Autodesk Fusion 360 part; units mm, degrees
(part 5 of 11)
  arc A140 (-29.854, -24.6972) -> (-30.0927, -24.4471) centre (-30.104, -24.6968) ccw construction
  arc A141 (-29.854, -24.6972) -> (-29.853, -24.8125) centre (-23.9648, -24.7074) ccw construction
  arc A142 (-30.0877, -25.0665) -> (-29.853, -24.8125) centre (-30.103, -24.8169) ccw construction
  line L76 (-30.0877, -25.0665) -> (-30.1561, -25.0707) construction
  spline S70 degree 5 poles (-30.1561, -25.0707) (-30.1588, -25.0708) (-30.1643, -25.0712) (-30.1725, -25.072) (-30.1834, -25.0735) (-30.197, -25.0758) (-30.2105, -25.0785) (-30.224, -25.0814) (-30.2375, -25.0845) (-30.251, -25.0877) (-30.2645, -25.091) (-30.278, -25.0944) (-30.2915, -25.098) (-30.3049, -25.1017) (-30.3183, -25.1056) (-30.3317, -25.1097) (-30.3451, -25.114) (-30.3585, -25.1183) (-30.3719, -25.1228) (-30.3852, -25.1274) (-30.3986, -25.1321) (-30.4119, -25.1369) (-30.4252, -25.1418) (-30.4385, -25.1469) (-30.4518, -25.152) (-30.4651, -25.1573) (-30.4783, -25.1626) (-30.4915, -25.1681) (-30.5048, -25.1737) (-30.518, -25.1793) (-30.5312, -25.1851) (-30.5443, -25.1909) (-30.5575, -25.1969) (-30.5707, -25.2029) (-30.5838, -25.2091) (-30.5969, -25.2153) (-30.61, -25.2216) (-30.6231, -25.228) (-30.6362, -25.2345) (-30.6492, -25.2411) (-30.6623, -25.2478) (-30.6753, -25.2545) (-30.6883, -25.2613) (-30.7013, -25.2683) (-30.7143, -25.2753) (-30.7272, -25.2824) (-30.7402, -25.2895) (-30.7531, -25.2968) (-30.766, -25.3041) (-30.7789, -25.3115) (-30.7918, -25.319) (-30.8046, -25.3266) (-30.8175, -25.3342) (-30.8303, -25.3419) (-30.8431, -25.3497) (-30.8559, -25.3576) (-30.8686, -25.3655) (-30.8814, -25.3735) (-30.8941, -25.3816) (-30.9068, -25.3898) (-30.9195, -25.398) (-30.9322, -25.4064) (-30.9449, -25.4147) (-30.9575, -25.4232) (-30.9701, -25.4317) (-30.9827, -25.4403) (-30.9953, -25.449) (-31.0079, -25.4578) (-31.0204, -25.4666) (-31.033, -25.4755) (-31.0455, -25.4844) (-31.0555, -25.4916) (-31.0629, -25.4971) (-31.0679, -25.5007) (-31.0704, -25.5025) knots 0 0 0 0 0 0 0.01428571 0.02857143 0.04285714 0.05714286 0.07142857 0.08571429 0.1 0.11428571 0.12857143 0.14285714 0.15714286 0.17142857 0.18571429 0.2 0.21428571 0.22857143 0.24285714 0.25714286 0.27142857 0.28571429 0.3 0.31428571 0.32857143 0.34285714 0.35714286 0.37142857 0.38571429 0.4 0.41428571 0.42857143 0.44285714 0.45714286 0.47142857 0.48571429 0.5 0.51428571 0.52857143 0.54285714 0.55714286 0.57142857 0.58571429 0.6 0.61428571 0.62857143 0.64285714 0.65714286 0.67142857 0.68571429 0.7 0.71428571 0.72857143 0.74285714 0.75714286 0.77142857 0.78571429 0.8 0.81428571 0.82857143 0.84285714 0.85714286 0.87142857 0.88571429 0.9 0.91428571 0.92857143 0.94285714 0.95714286 0.97142857 0.98571429 1 1 1 1 1 1 construction
  arc A143 (-31.0704, -25.5025) -> (-31.0159, -25.8922) centre (-23.9648, -24.7074) ccw construction
  spline S71 degree 5 poles (-31.0159, -25.8922) (-31.013, -25.8933) (-31.0072, -25.8955) (-30.9985, -25.8986) (-30.9869, -25.9028) (-30.9725, -25.908) (-30.958, -25.9131) (-30.9435, -25.9182) (-30.929, -25.9231) (-30.9145, -25.928) (-30.9001, -25.9328) (-30.8856, -25.9376) (-30.8711, -25.9422) (-30.8566, -25.9468) (-30.8422, -25.9513) (-30.8277, -25.9558) (-30.8132, -25.9601) (-30.7988, -25.9644) (-30.7843, -25.9687) (-30.7698, -25.9728) (-30.7554, -25.9768) (-30.7409, -25.9808) (-30.7265, -25.9847) (-30.712, -25.9886) (-30.6976, -25.9923) (-30.6832, -25.996) (-30.6687, -25.9996) (-30.6543, -26.0031) (-30.6399, -26.0065) (-30.6255, -26.0098) (-30.6111, -26.0131) (-30.5967, -26.0163) (-30.5823, -26.0193) (-30.5679, -26.0223) (-30.5535, -26.0253) (-30.5392, -26.0281) (-30.5248, -26.0308) (-30.5104, -26.0335) (-30.4961, -26.0361) (-30.4818, -26.0386) (-30.4674, -26.0409) (-30.4531, -26.0432) (-30.4388, -26.0454) (-30.4245, -26.0476) (-30.4103, -26.0496) (-30.396, -26.0515) (-30.3817, -26.0533) (-30.3675, -26.055) (-30.3533, -26.0567) (-30.3391, -26.0582) (-30.3249, -26.0596) (-30.3107, -26.0609) (-30.2965, -26.0621) (-30.2824, -26.0632) (-30.2682, -26.0641) (-30.2541, -26.065) (-30.24, -26.0657) (-30.2259, -26.0664) (-30.2119, -26.0669) (-30.1978, -26.0673) (-30.1838, -26.0676) (-30.1698, -26.0677) (-30.1558, -26.0676) (-30.1419, -26.0673) (-30.128, -26.0669) (-30.1141, -26.0663) (-30.1003, -26.0657) (-30.0865, -26.065) (-30.0727, -26.0641) (-30.0589, -26.063) (-30.0452, -26.0615) (-30.0343, -26.0599) (-30.0262, -26.0584) (-30.0209, -26.0573) (-30.0182, -26.0567) knots -1 -1 -1 -1 -1 -1 -0.98571429 -0.97142857 -0.95714286 -0.94285714 -0.92857143 -0.91428571 -0.9 -0.88571429 -0.87142857 -0.85714286 -0.84285714 -0.82857143 -0.81428571 -0.8 -0.78571429 -0.77142857 -0.75714286 -0.74285714 -0.72857143 -0.71428571 -0.7 -0.68571429 -0.67142857 -0.65714286 -0.64285714 -0.62857143 -0.61428571 -0.6 -0.58571429 -0.57142857 -0.55714286 -0.54285714 -0.52857143 -0.51428571 -0.5 -0.48571429 -0.47142857 -0.45714286 -0.44285714 -0.42857143 -0.41428571 -0.4 -0.38571429 -0.37142857 -0.35714286 -0.34285714 -0.32857143 -0.31428571 -0.3 -0.28571429 -0.27142857 -0.25714286 -0.24285714 -0.22857143 -0.21428571 -0.2 -0.18571429 -0.17142857 -0.15714286 -0.14285714 -0.12857143 -0.11428571 -0.1 -0.08571429 -0.07142857 -0.05714286 -0.04285714 -0.02857143 -0.01428571 0 0 0 0 0 0 construction
  line L77 (-30.0182, -26.0567) -> (-29.9513, -26.042) construction
  arc A144 (-29.6559, -26.2218) -> (-29.9513, -26.042) centre (-29.8975, -26.2861) ccw construction
  arc A145 (-29.6559, -26.2218) -> (-29.6252, -26.3329) centre (-23.9648, -24.7074) ccw construction
  arc A146 (-29.7862, -26.639) -> (-29.6252, -26.3329) centre (-29.8655, -26.4019) ccw construction
  line L78 (-29.7862, -26.639) -> (-29.8511, -26.6607) construction
  spline S72 degree 5 poles (-29.8511, -26.6607) (-29.8537, -26.6616) (-29.8589, -26.6634) (-29.8666, -26.6663) (-29.8768, -26.6705) (-29.8893, -26.6763) (-29.9016, -26.6824) (-29.9139, -26.6887) (-29.9262, -26.6952) (-29.9384, -26.7018) (-29.9506, -26.7084) (-29.9627, -26.7152) (-29.9748, -26.7221) (-29.9868, -26.7292) (-29.9988, -26.7365) (-30.0107, -26.7439) (-30.0225, -26.7515) (-30.0343, -26.7592) (-30.046, -26.767) (-30.0578, -26.7748) (-30.0694, -26.7828) (-30.0811, -26.7909) (-30.0926, -26.7991) (-30.1042, -26.8074) (-30.1157, -26.8158) (-30.1271, -26.8243) (-30.1385, -26.8329) (-30.1499, -26.8417) (-30.1612, -26.8505) (-30.1725, -26.8593) (-30.1838, -26.8683) (-30.195, -26.8774) (-30.2062, -26.8865) (-30.2173, -26.8958) (-30.2284, -26.9051) (-30.2395, -26.9145) (-30.2505, -26.924) (-30.2615, -26.9336) (-30.2724, -26.9432) (-30.2833, -26.953) (-30.2942, -26.9628) (-30.305, -26.9727) (-30.3158, -26.9826) (-30.3266, -26.9927) (-30.3373, -27.0028) (-30.348, -27.013) (-30.3586, -27.0233) (-30.3692, -27.0336) (-30.3798, -27.0441) (-30.3904, -27.0545) (-30.4009, -27.0651) (-30.4113, -27.0757) (-30.4217, -27.0864) (-30.4321, -27.0972) (-30.4425, -27.1081) (-30.4528, -27.119) (-30.4631, -27.1299) (-30.4733, -27.141) (-30.4835, -27.1521) (-30.4937, -27.1633) (-30.5038, -27.1745) (-30.5139, -27.1859) (-30.524, -27.1972) (-30.534, -27.2087) (-30.544, -27.2202) (-30.5539, -27.2318) (-30.5638, -27.2434) (-30.5737, -27.2551) (-30.5835, -27.2668) (-30.5933, -27.2787) (-30.6031, -27.2906) (-30.6109, -27.3001) (-30.6167, -27.3073) (-30.6206, -27.3121) (-30.6225, -27.3145) knots 0 0 0 0 0 0 0.01428571 0.02857143 0.04285714 0.05714286 0.07142857 0.08571429 0.1 0.11428571 0.12857143 0.14285714 0.15714286 0.17142857 0.18571429 0.2 0.21428571 0.22857143 0.24285714 0.25714286 0.27142857 0.28571429 0.3 0.31428571 0.32857143 0.34285714 0.35714286 0.37142857 0.38571429 0.4 0.41428571 0.42857143 0.44285714 0.45714286 0.47142857 0.48571429 0.5 0.51428571 0.52857143 0.54285714 0.55714286 0.57142857 0.58571429 0.6 0.61428571 0.62857143 0.64285714 0.65714286 0.67142857 0.68571429 0.7 0.71428571 0.72857143 0.74285714 0.75714286 0.77142857 0.78571429 0.8 0.81428571 0.82857143 0.84285714 0.85714286 0.87142857 0.88571429 0.9 0.91428571 0.92857143 0.94285714 0.95714286 0.97142857 0.98571429 1 1 1 1 1 1 construction
  arc A147 (-30.6225, -27.3145) -> (-30.469, -27.6768) centre (-23.9648, -24.7074) ccw construction
  spline S73 degree 5 poles (-30.469, -27.6768) (-30.4659, -27.6771) (-30.4598, -27.6777) (-30.4505, -27.6785) (-30.4383, -27.6796) (-30.4229, -27.6808) (-30.4076, -27.682) (-30.3923, -27.6831) (-30.3771, -27.6842) (-30.3618, -27.6851) (-30.3466, -27.6861) (-30.3314, -27.6869) (-30.3162, -27.6876) (-30.301, -27.6883) (-30.2859, -27.689) (-30.2707, -27.6895) (-30.2556, -27.69) (-30.2405, -27.6904) (-30.2255, -27.6907) (-30.2104, -27.691) (-30.1954, -27.6911) (-30.1804, -27.6912) (-30.1655, -27.6913) (-30.1505, -27.6912) (-30.1356, -27.6911) (-30.1207, -27.6909) (-30.1059, -27.6906) (-30.091, -27.6903) (-30.0762, -27.6899) (-30.0614, -27.6894) (-30.0467, -27.6888) (-30.0319, -27.6881) (-30.0172, -27.6874) (-30.0026, -27.6866) (-29.9879, -27.6857) (-29.9733, -27.6847) (-29.9587, -27.6836) (-29.9442, -27.6825) (-29.9297, -27.6812) (-29.9152, -27.6799) (-29.9007, -27.6785) (-29.8863, -27.677) (-29.8719, -27.6755) (-29.8576, -27.6738) (-29.8433, -27.6721) (-29.829, -27.6702) (-29.8147, -27.6683) (-29.8005, -27.6663) (-29.7864, -27.6642) (-29.7722, -27.6619) (-29.7582, -27.6596) (-29.7441, -27.6572) (-29.7301, -27.6547) (-29.7162, -27.6521) (-29.7023, -27.6494) (-29.6884, -27.6465) (-29.6746, -27.6436) (-29.6608, -27.6406) (-29.6471, -27.6375) (-29.6334, -27.6342) (-29.6198, -27.6308) (-29.6063, -27.6273) (-29.5928, -27.6236) (-29.5795, -27.6197) (-29.5661, -27.6157) (-29.5529, -27.6116) (-29.5397, -27.6074) (-29.5265, -27.6031) (-29.5134, -27.5987) (-29.5004, -27.5941) (-29.4876, -27.5891) (-29.4775, -27.5847) (-29.47, -27.5812) (-29.4651, -27.5787) (-29.4627, -27.5775) knots -1 -1 -1 -1 -1 -1 -0.98571429 -0.97142857 -0.95714286 -0.94285714 -0.92857143 -0.91428571 -0.9 -0.88571429 -0.87142857 -0.85714286 -0.84285714 -0.82857143 -0.81428571 -0.8 -0.78571429 -0.77142857 -0.75714286 -0.74285714 -0.72857143 -0.71428571 -0.7 -0.68571429 -0.67142857 -0.65714286 -0.64285714 -0.62857143 -0.61428571 -0.6 -0.58571429 -0.57142857 -0.55714286 -0.54285714 -0.52857143 -0.51428571 -0.5 -0.48571429 -0.47142857 -0.45714286 -0.44285714 -0.42857143 -0.41428571 -0.4 -0.38571429 -0.37142857 -0.35714286 -0.34285714 -0.32857143 -0.31428571 -0.3 -0.28571429 -0.27142857 -0.25714286 -0.24285714 -0.22857143 -0.21428571 -0.2 -0.18571429 -0.17142857 -0.15714286 -0.14285714 -0.12857143 -0.11428571 -0.1 -0.08571429 -0.07142857 -0.05714286 -0.04285714 -0.02857143 -0.01428571 0 0 0 0 0 0 construction
  line L79 (-29.4627, -27.5775) -> (-29.4019, -27.5459) construction
  arc A148 (-29.07, -27.6432) -> (-29.4019, -27.5459) centre (-29.2868, -27.7678) ccw construction
  arc A149 (-29.07, -27.6432) -> (-29.0116, -27.7425) centre (-23.9648, -24.7074) ccw construction
  arc A150 (-29.0879, -28.0799) -> (-29.0116, -27.7425) centre (-29.2258, -27.8714) ccw construction
  line L80 (-29.0879, -28.0799) -> (-29.145, -28.1177) construction
  spline S74 degree 5 poles (-29.145, -28.1177) (-29.1473, -28.1192) (-29.1518, -28.1223) (-29.1585, -28.1271) (-29.1672, -28.1337) (-29.1778, -28.1425) (-29.1882, -28.1516) (-29.1984, -28.161) (-29.2086, -28.1704) (-29.2186, -28.1799) (-29.2287, -28.1895) (-29.2387, -28.1992) (-29.2486, -28.209) (-29.2583, -28.2189) (-29.268, -28.2291) (-29.2776, -28.2393) (-29.287, -28.2497) (-29.2964, -28.2602) (-29.3058, -28.2707) (-29.315, -28.2814) (-29.3242, -28.2921) (-29.3334, -28.3029) (-29.3425, -28.3138) (-29.3515, -28.3249) (-29.3604, -28.336) (-29.3693, -28.3471) (-29.378, -28.3584) (-29.3868, -28.3698) (-29.3954, -28.3812) (-29.404, -28.3927) (-29.4126, -28.4043) (-29.4211, -28.4159) (-29.4295, -28.4277) (-29.4379, -28.4395) (-29.4462, -28.4514) (-29.4544, -28.4633) (-29.4626, -28.4753) (-29.4707, -28.4874) (-29.4788, -28.4996) (-29.4868, -28.5118) (-29.4948, -28.5241) (-29.5027, -28.5365) (-29.5105, -28.5489) (-29.5183, -28.5614) (-29.5261, -28.5739) (-29.5337, -28.5866) (-29.5414, -28.5992) (-29.5489, -28.612) (-29.5565, -28.6248) (-29.5639, -28.6376) (-29.5713, -28.6505) (-29.5787, -28.6635) (-29.586, -28.6766) (-29.5932, -28.6897) (-29.6004, -28.7028) (-29.6076, -28.716) (-29.6146, -28.7293) (-29.6217, -28.7426) (-29.6287, -28.756) (-29.6356, -28.7694) (-29.6425, -28.7829) (-29.6493, -28.7964) (-29.656, -28.81) (-29.6628, -28.8237) (-29.6694, -28.8374) (-29.676, -28.8511) (-29.6826, -28.8649) (-29.6891, -28.8788) (-29.6956, -28.8927) (-29.702, -28.9067) (-29.7083, -28.9207) (-29.7134, -28.9319) (-29.7171, -28.9404) (-29.7196, -28.946) (-29.7209, -28.9488) knots 0 0 0 0 0 0 0.01428571 0.02857143 0.04285714 0.05714286 0.07142857 0.08571429 0.1 0.11428571 0.12857143 0.14285714 0.15714286 0.17142857 0.18571429 0.2 0.21428571 0.22857143 0.24285714 0.25714286 0.27142857 0.28571429 0.3 0.31428571 0.32857143 0.34285714 0.35714286 0.37142857 0.38571429 0.4 0.41428571 0.42857143 0.44285714 0.45714286 0.47142857 0.48571429 0.5 0.51428571 0.52857143 0.54285714 0.55714286 0.57142857 0.58571429 0.6 0.61428571 0.62857143 0.64285714 0.65714286 0.67142857 0.68571429 0.7 0.71428571 0.72857143 0.74285714 0.75714286 0.77142857 0.78571429 0.8 0.81428571 0.82857143 0.84285714 0.85714286 0.87142857 0.88571429 0.9 0.91428571 0.92857143 0.94285714 0.95714286 0.97142857 0.98571429 1 1 1 1 1 1 construction
  arc A151 (-29.7209, -28.9488) -> (-29.4788, -29.2591) centre (-23.9648, -24.7074) ccw construction
  spline S75 degree 5 poles (-29.4788, -29.2591) (-29.4758, -29.2586) (-29.4697, -29.2575) (-29.4606, -29.2559) (-29.4484, -29.2538) (-29.4333, -29.251) (-29.4182, -29.2482) (-29.4032, -29.2453) (-29.3881, -29.2424) (-29.3731, -29.2394) (-29.3582, -29.2363) (-29.3433, -29.2332) (-29.3284, -29.23) (-29.3136, -29.2267) (-29.2988, -29.2234) (-29.284, -29.22) (-29.2693, -29.2165) (-29.2547, -29.213) (-29.24, -29.2094) (-29.2254, -29.2058) (-29.2109, -29.2021) (-29.1964, -29.1983) (-29.1819, -29.1945) (-29.1675, -29.1905) (-29.1531, -29.1866) (-29.1388, -29.1825) (-29.1245, -29.1784) (-29.1103, -29.1742) (-29.0961, -29.17) (-29.0819, -29.1657) (-29.0678, -29.1613) (-29.0537, -29.1569) (-29.0397, -29.1523) (-29.0258, -29.1477) (-29.0119, -29.1431) (-28.998, -29.1384) (-28.9842, -29.1336) (-28.9704, -29.1287) (-28.9567, -29.1237) (-28.9431, -29.1187) (-28.9295, -29.1136) (-28.9159, -29.1085) (-28.9024, -29.1032) (-28.889, -29.0979) (-28.8756, -29.0925) (-28.8623, -29.087) (-28.8491, -29.0815) (-28.8359, -29.0758) (-28.8227, -29.0701) (-28.8097, -29.0644) (-28.7967, -29.0585) (-28.7837, -29.0525) (-28.7709, -29.0465) (-28.7581, -29.0403) (-28.7453, -29.0341) (-28.7327, -29.0278) (-28.7201, -29.0214) (-28.7076, -29.0149) (-28.6951, -29.0083) (-28.6828, -29.0017) (-28.6705, -28.9949) (-28.6583, -28.988) (-28.6463, -28.9809) (-28.6344, -28.9737) (-28.6226, -28.9664) (-28.6108, -28.959) (-28.5991, -28.9515) (-28.5875, -28.9439) (-28.576, -28.9363) (-28.5647, -28.9284) (-28.5535, -28.9203) (-28.5449, -28.9135) (-28.5387, -28.9081) (-28.5346, -28.9045) (-28.5325, -28.9026) knots -1 -1 -1 -1 -1 -1 -0.98571429 -0.97142857 -0.95714286 -0.94285714 -0.92857143 -0.91428571 -0.9 -0.88571429 -0.87142857 -0.85714286 -0.84285714 -0.82857143 -0.81428571 -0.8 -0.78571429 -0.77142857 -0.75714286 -0.74285714 -0.72857143 -0.71428571 -0.7 -0.68571429 -0.67142857 -0.65714286 -0.64285714 -0.62857143 -0.61428571 -0.6 -0.58571429 -0.57142857 -0.55714286 -0.54285714 -0.52857143 -0.51428571 -0.5 -0.48571429 -0.47142857 -0.45714286 -0.44285714 -0.42857143 -0.41428571 -0.4 -0.38571429 -0.37142857 -0.35714286 -0.34285714 -0.32857143 -0.31428571 -0.3 -0.28571429 -0.27142857 -0.25714286 -0.24285714 -0.22857143 -0.21428571 -0.2 -0.18571429 -0.17142857 -0.15714286 -0.14285714 -0.12857143 -0.11428571 -0.1 -0.08571429 -0.07142857 -0.05714286 -0.04285714 -0.02857143 -0.01428571 0 0 0 0 0 0 construction
  line L81 (-28.5325, -28.9026) -> (-28.482, -28.8564) construction
  arc A152 (-28.1362, -28.8645) -> (-28.482, -28.8564) centre (-28.3133, -29.041) ccw construction
  arc A153 (-28.1362, -28.8645) -> (-28.0541, -28.9453) centre (-23.9648, -24.7074) ccw construction
  arc A154 (-28.0404, -29.2909) -> (-28.0541, -28.9453) centre (-28.2277, -29.1252) ccw construction
  line L82 (-28.0404, -29.2909) -> (-28.0858, -29.3422) construction
  spline S76 degree 5 poles (-28.0858, -29.3422) (-28.0876, -29.3442) (-28.0912, -29.3484) (-28.0965, -29.3548) (-28.1032, -29.3635) (-28.1111, -29.3747) (-28.1188, -29.3862) (-28.1262, -29.3978) (-28.1336, -29.4096) (-28.1409, -29.4214) (-28.1481, -29.4332) (-28.1552, -29.4452) (-28.1622, -29.4572) (-28.1691, -29.4694) (-28.1758, -29.4816) (-28.1824, -29.494) (-28.1889, -29.5065) (-28.1952, -29.519) (-28.2015, -29.5317) (-28.2077, -29.5443) (-28.2138, -29.5571) (-28.2199, -29.5699) (-28.2258, -29.5828) (-28.2316, -29.5958) (-28.2374, -29.6088) (-28.2431, -29.6219) (-28.2486, -29.6351) (-28.2541, -29.6483) (-28.2595, -29.6616) (-28.2649, -29.6749) (-28.2701, -29.6883) (-28.2753, -29.7018) (-28.2804, -29.7153) (-28.2854, -29.7289) (-28.2904, -29.7425) (-28.2953, -29.7562) (-28.3001, -29.7699) (-28.3048, -29.7837) (-28.3094, -29.7975) (-28.314, -29.8114) (-28.3185, -29.8253) (-28.323, -29.8393) (-28.3273, -29.8534) (-28.3316, -29.8674) (-28.3358, -29.8816) (-28.34, -29.8957) (-28.3441, -29.91) (-28.3481, -29.9242) (-28.352, -29.9385) (-28.3559, -29.9529) (-28.3597, -29.9673) (-28.3635, -29.9817) (-28.3671, -29.9962) (-28.3708, -30.0107) (-28.3743, -30.0253) (-28.3778, -30.0399) (-28.3812, -30.0545) (-28.3845, -30.0692) (-28.3878, -30.084) (-28.391, -30.0987) (-28.3942, -30.1135) (-28.3973, -30.1284) (-28.4003, -30.1433) (-28.4032, -30.1582) (-28.4061, -30.1731) (-28.409, -30.1881) (-28.4117, -30.2032) (-28.4144, -30.2182) (-28.4171, -30.2333) (-28.4196, -30.2485) (-28.4222, -30.2636) (-28.4241, -30.2758) (-28.4256, -30.2849) (-28.4265, -30.291) (-28.427, -30.2941) knots 0 0 0 0 0 0 0.01428571 0.02857143 0.04285714 0.05714286 0.07142857 0.08571429 0.1 0.11428571 0.12857143 0.14285714 0.15714286 0.17142857 0.18571429 0.2 0.21428571 0.22857143 0.24285714 0.25714286 0.27142857 0.28571429 0.3 0.31428571 0.32857143 0.34285714 0.35714286 0.37142857 0.38571429 0.4 0.41428571 0.42857143 0.44285714 0.45714286 0.47142857 0.48571429 0.5 0.51428571 0.52857143 0.54285714 0.55714286 0.57142857 0.58571429 0.6 0.61428571 0.62857143 0.64285714 0.65714286 0.67142857 0.68571429 0.7 0.71428571 0.72857143 0.74285714 0.75714286 0.77142857 0.78571429 0.8 0.81428571 0.82857143 0.84285714 0.85714286 0.87142857 0.88571429 0.9 0.91428571 0.92857143 0.94285714 0.95714286 0.97142857 0.98571429 1 1 1 1 1 1 construction
  arc A155 (-28.427, -30.2941) -> (-28.1129, -30.5311) centre (-23.9648, -24.7074) ccw construction
  spline S77 degree 5 poles (-28.1129, -30.5311) (-28.1101, -30.5298) (-28.1045, -30.5272) (-28.0961, -30.5234) (-28.0849, -30.5181) (-28.071, -30.5116) (-28.0571, -30.5049) (-28.0433, -30.4982) (-28.0296, -30.4915) (-28.0159, -30.4847) (-28.0023, -30.4779) (-27.9887, -30.471) (-27.9751, -30.4641) (-27.9616, -30.4571) (-27.9482, -30.45) (-27.9348, -30.443) (-27.9215, -30.4358) (-27.9083, -30.4286) (-27.8951, -30.4214) (-27.8819, -30.4141) (-27.8688, -30.4067) (-27.8558, -30.3993) (-27.8428, -30.3919) (-27.8299, -30.3844) (-27.817, -30.3768) (-27.8042, -30.3692) (-27.7915, -30.3615) (-27.7788, -30.3538) (-27.7662, -30.346) (-27.7536, -30.3382) (-27.7412, -30.3303) (-27.7287, -30.3224) (-27.7164, -30.3144) (-27.7041, -30.3063) (-27.6918, -30.2982) (-27.6797, -30.2901) (-27.6676, -30.2819) (-27.6556, -30.2736) (-27.6436, -30.2653) (-27.6317, -30.2569) (-27.6199, -30.2485) (-27.6081, -30.24) (-27.5965, -30.2314) (-27.5849, -30.2228) (-27.5734, -30.2141) (-27.5619, -30.2054) (-27.5506, -30.1966) (-27.5393, -30.1877) (-27.528, -30.1788) (-27.5169, -30.1699) (-27.5059, -30.1608) (-27.4949, -30.1517) (-27.4841, -30.1425) (-27.4733, -30.1333) (-27.4626, -30.124) (-27.452, -30.1146) (-27.4415, -30.1052) (-27.4311, -30.0957) (-27.4208, -30.0861) (-27.4106, -30.0764) (-27.4005, -30.0667) (-27.3905, -30.0569) (-27.3807, -30.0469) (-27.3711, -30.0369) (-27.3615, -30.0268) (-27.3521, -30.0166) (-27.3428, -30.0063) (-27.3335, -29.996) (-27.3244, -29.9857) (-27.3154, -29.9751) (-27.3068, -29.9644) (-27.3003, -29.9556) (-27.2956, -29.9488) (-27.2926, -29.9442) (-27.2911, -29.9419) knots -1 -1 -1 -1 -1 -1 -0.98571429 -0.97142857 -0.95714286 -0.94285714 -0.92857143 -0.91428571 -0.9 -0.88571429 -0.87142857 -0.85714286 -0.84285714 -0.82857143 -0.81428571 -0.8 -0.78571429 -0.77142857 -0.75714286 -0.74285714 -0.72857143 -0.71428571 -0.7 -0.68571429 -0.67142857 -0.65714286 -0.64285714 -0.62857143 -0.61428571 -0.6 -0.58571429 -0.57142857 -0.55714286 -0.54285714 -0.52857143 -0.51428571 -0.5 -0.48571429 -0.47142857 -0.45714286 -0.44285714 -0.42857143 -0.41428571 -0.4 -0.38571429 -0.37142857 -0.35714286 -0.34285714 -0.32857143 -0.31428571 -0.3 -0.28571429 -0.27142857 -0.25714286 -0.24285714 -0.22857143 -0.21428571 -0.2 -0.18571429 -0.17142857 -0.15714286 -0.14285714 -0.12857143 -0.11428571 -0.1 -0.08571429 -0.07142857 -0.05714286 -0.04285714 -0.02857143 -0.01428571 0 0 0 0 0 0 construction
  line L83 (-27.2911, -29.9419) -> (-27.2542, -29.8842) construction
  arc A156 (-26.9182, -29.8025) -> (-27.2542, -29.8842) centre (-27.0435, -30.0188) ccw construction
  arc A157 (-26.9182, -29.8025) -> (-26.8179, -29.8593) centre (-23.9648, -24.7074) ccw construction
  arc A158 (-26.7153, -30.1896) -> (-26.8179, -29.8593) centre (-26.939, -30.078) ccw construction
  line L84 (-26.7153, -30.1896) -> (-26.7458, -30.2509) construction
  spline S78 degree 5 poles (-26.7458, -30.2509) (-26.7471, -30.2533) (-26.7495, -30.2583) (-26.7529, -30.2658) (-26.7571, -30.2759) (-26.7618, -30.2888) (-26.7662, -30.3019) (-26.7704, -30.3151) (-26.7745, -30.3283) (-26.7785, -30.3416) (-26.7824, -30.3549) (-26.7862, -30.3683) (-26.7899, -30.3818) (-26.7934, -30.3953) (-26.7967, -30.4089) (-26.7998, -30.4225) (-26.8029, -30.4362) (-26.8058, -30.45) (-26.8086, -30.4638) (-26.8113, -30.4777) (-26.8139, -30.4916) (-26.8164, -30.5055) (-26.8188, -30.5195) (-26.8211, -30.5336) (-26.8232, -30.5476) (-26.8253, -30.5617) (-26.8273, -30.5759) (-26.8292, -30.5901) (-26.831, -30.6043) (-26.8327, -30.6186) (-26.8343, -30.6329) (-26.8358, -30.6473) (-26.8372, -30.6616) (-26.8386, -30.676) (-26.8398, -30.6905) (-26.841, -30.705) (-26.8421, -30.7195) (-26.8431, -30.734) (-26.844, -30.7486) (-26.8448, -30.7632) (-26.8456, -30.7778) (-26.8462, -30.7924) (-26.8468, -30.8071) (-26.8473, -30.8218) (-26.8477, -30.8366) (-26.8481, -30.8513) (-26.8483, -30.8661) (-26.8485, -30.8809) (-26.8486, -30.8958) (-26.8487, -30.9107) (-26.8486, -30.9255) (-26.8485, -30.9405) (-26.8483, -30.9554) (-26.848, -30.9704) (-26.8477, -30.9854) (-26.8473, -31.0004) (-26.8468, -31.0154) (-26.8462, -31.0304) (-26.8455, -31.0455) (-26.8448, -31.0606) (-26.844, -31.0757) (-26.8432, -31.0909) (-26.8422, -31.106) (-26.8412, -31.1212) (-26.8402, -31.1364) (-26.839, -31.1516) (-26.8378, -31.1669) (-26.8365, -31.1821) (-26.8351, -31.1974) (-26.8337, -31.2127) (-26.8322, -31.228) (-26.831, -31.2402) (-26.83, -31.2494) (-26.8293, -31.2556) (-26.829, -31.2586) knots 0 0 0 0 0 0 0.01428571 0.02857143 0.04285714 0.05714286 0.07142857 0.08571429 0.1 0.11428571 0.12857143 0.14285714 0.15714286 0.17142857 0.18571429 0.2 0.21428571 0.22857143 0.24285714 0.25714286 0.27142857 0.28571429 0.3 0.31428571 0.32857143 0.34285714 0.35714286 0.37142857 0.38571429 0.4 0.41428571 0.42857143 0.44285714 0.45714286 0.47142857 0.48571429 0.5 0.51428571 0.52857143 0.54285714 0.55714286 0.57142857 0.58571429 0.6 0.61428571 0.62857143 0.64285714 0.65714286 0.67142857 0.68571429 0.7 0.71428571 0.72857143 0.74285714 0.75714286 0.77142857 0.78571429 0.8 0.81428571 0.82857143 0.84285714 0.85714286 0.87142857 0.88571429 0.9 0.91428571 0.92857143 0.94285714 0.95714286 0.97142857 0.98571429 1 1 1 1 1 1 construction
  arc A159 (-26.829, -31.2586) -> (-26.4642, -31.4063) centre (-23.9648, -24.7074) ccw construction
  spline S79 degree 5 poles (-26.4642, -31.4063) (-26.4619, -31.4043) (-26.4571, -31.4004) (-26.45, -31.3944) (-26.4406, -31.3865) (-26.4289, -31.3766) (-26.4172, -31.3666) (-26.4056, -31.3565) (-26.3941, -31.3465) (-26.3826, -31.3364) (-26.3712, -31.3263) (-26.3598, -31.3161) (-26.3485, -31.3059) (-26.3373, -31.2956) (-26.3262, -31.2854) (-26.3151, -31.2751) (-26.3041, -31.2647) (-26.2931, -31.2543) (-26.2823, -31.2439) (-26.2714, -31.2335) (-26.2607, -31.223) (-26.25, -31.2124) (-26.2394, -31.2019) (-26.2289, -31.1913) (-26.2184, -31.1807) (-26.208, -31.17) (-26.1977, -31.1593) (-26.1875, -31.1485) (-26.1773, -31.1378) (-26.1672, -31.127) (-26.1572, -31.1161) (-26.1472, -31.1052) (-26.1373, -31.0943) (-26.1276, -31.0834) (-26.1178, -31.0724) (-26.1082, -31.0613) (-26.0986, -31.0503) (-26.0892, -31.0392) (-26.0798, -31.028) (-26.0704, -31.0169) (-26.0612, -31.0057) (-26.0521, -30.9944) (-26.043, -30.9831) (-26.034, -30.9718) (-26.0252, -30.9604) (-26.0164, -30.949) (-26.0077, -30.9376) (-25.999, -30.9261) (-25.9905, -30.9146) (-25.9821, -30.9031) (-25.9738, -30.8915) (-25.9655, -30.8799) (-25.9574, -30.8682) (-25.9494, -30.8565) (-25.9415, -30.8447) (-25.9337, -30.8329) (-25.926, -30.8211) (-25.9184, -30.8092) (-25.9109, -30.7973) (-25.9035, -30.7853) (-25.8963, -30.7733) (-25.8892, -30.7613) (-25.8823, -30.7491) (-25.8756, -30.7369) (-25.869, -30.7247) (-25.8626, -30.7124) (-25.8562, -30.7001) (-25.8499, -30.6877) (-25.8438, -30.6753) (-25.8379, -30.6629) (-25.8323, -30.6503) (-25.8283, -30.6401) (-25.8255, -30.6323) (-25.8238, -30.6271) (-25.8229, -30.6245) knots -1 -1 -1 -1 -1 -1 -0.98571429 -0.97142857 -0.95714286 -0.94285714 -0.92857143 -0.91428571 -0.9 -0.88571429 -0.87142857 -0.85714286 -0.84285714 -0.82857143 -0.81428571 -0.8 -0.78571429 -0.77142857 -0.75714286 -0.74285714 -0.72857143 -0.71428571 -0.7 -0.68571429 -0.67142857 -0.65714286 -0.64285714 -0.62857143 -0.61428571 -0.6 -0.58571429 -0.57142857 -0.55714286 -0.54285714 -0.52857143 -0.51428571 -0.5 -0.48571429 -0.47142857 -0.45714286 -0.44285714 -0.42857143 -0.41428571 -0.4 -0.38571429 -0.37142857 -0.35714286 -0.34285714 -0.32857143 -0.31428571 -0.3 -0.28571429 -0.27142857 -0.25714286 -0.24285714 -0.22857143 -0.21428571 -0.2 -0.18571429 -0.17142857 -0.15714286 -0.14285714 -0.12857143 -0.11428571 -0.1 -0.08571429 -0.07142857 -0.05714286 -0.04285714 -0.02857143 -0.01428571 0 0 0 0 0 0 construction
  line L85 (-25.8229, -30.6245) -> (-25.8023, -30.5592) construction
  arc A160 (-25.4988, -30.3933) -> (-25.8023, -30.5592) centre (-25.5639, -30.6347) ccw construction
  arc A161 (-25.4988, -30.3933) -> (-25.3873, -30.4222) centre (-23.9648, -24.7074) ccw construction
  arc A162 (-25.2027, -30.7147) -> (-25.3873, -30.4222) centre (-25.4476, -30.6648) ccw construction
  line L86 (-25.2027, -30.7147) -> (-25.2163, -30.7818) construction
  spline S80 degree 5 poles (-25.2163, -30.7818) (-25.2169, -30.7845) (-25.2179, -30.7899) (-25.2192, -30.798) (-25.2207, -30.8089) (-25.2219, -30.8226) (-25.2228, -30.8364) (-25.2235, -30.8502) (-25.224, -30.864) (-25.2244, -30.8779) (-25.2247, -30.8918) (-25.2249, -30.9057) (-25.225, -30.9196) (-25.2249, -30.9336) (-25.2245, -30.9475) (-25.2241, -30.9616) (-25.2234, -30.9756) (-25.2227, -30.9896) (-25.2218, -31.0037) (-25.2208, -31.0178) (-25.2197, -31.0319) (-25.2185, -31.046) (-25.2172, -31.0601) (-25.2158, -31.0743) (-25.2143, -31.0885) (-25.2126, -31.1026) (-25.2109, -31.1168) (-25.209, -31.131) (-25.2071, -31.1452) (-25.205, -31.1595) (-25.2029, -31.1737) (-25.2006, -31.1879) (-25.1983, -31.2022) (-25.1959, -31.2165) (-25.1933, -31.2307) (-25.1907, -31.245) (-25.188, -31.2593) (-25.1852, -31.2736) (-25.1823, -31.2879) (-25.1793, -31.3022) (-25.1763, -31.3165) (-25.1731, -31.3309) (-25.1699, -31.3452) (-25.1665, -31.3595) (-25.1631, -31.3739) (-25.1597, -31.3882) (-25.1561, -31.4026) (-25.1524, -31.417) (-25.1487, -31.4313) (-25.1449, -31.4457) (-25.141, -31.4601) (-25.137, -31.4744) (-25.1329, -31.4888) (-25.1288, -31.5032) (-25.1246, -31.5176) (-25.1203, -31.532) (-25.1159, -31.5464) (-25.1115, -31.5608) (-25.107, -31.5752) (-25.1024, -31.5896) (-25.0977, -31.6039) (-25.0929, -31.6183) (-25.0881, -31.6327) (-25.0832, -31.6471) (-25.0782, -31.6615) (-25.0732, -31.6759) (-25.0681, -31.6903) (-25.0629, -31.7047) (-25.0576, -31.7191) (-25.0523, -31.7335) (-25.0469, -31.7479) (-25.0425, -31.7595) (-25.0391, -31.7681) (-25.0369, -31.7738) (-25.0358, -31.7767) knots 0 0 0 0 0 0 0.01428571 0.02857143 0.04285714 0.05714286 0.07142857 0.08571429 0.1 0.11428571 0.12857143 0.14285714 0.15714286 0.17142857 0.18571429 0.2 0.21428571 0.22857143 0.24285714 0.25714286 0.27142857 0.28571429 0.3 0.31428571 0.32857143 0.34285714 0.35714286 0.37142857 0.38571429 0.4 0.41428571 0.42857143 0.44285714 0.45714286 0.47142857 0.48571429 0.5 0.51428571 0.52857143 0.54285714 0.55714286 0.57142857 0.58571429 0.6 0.61428571 0.62857143 0.64285714 0.65714286 0.67142857 0.68571429 0.7 0.71428571 0.72857143 0.74285714 0.75714286 0.77142857 0.78571429 0.8 0.81428571 0.82857143 0.84285714 0.85714286 0.87142857 0.88571429 0.9 0.91428571 0.92857143 0.94285714 0.95714286 0.97142857 0.98571429 1 1 1 1 1 1 construction
  arc A163 (-25.0358, -31.7767) -> (-24.6453, -31.8249) centre (-23.9648, -24.7074) ccw construction
  spline S81 degree 5 poles (-24.6453, -31.8249) (-24.6435, -31.8224) (-24.6399, -31.8174) (-24.6346, -31.8098) (-24.6275, -31.7997) (-24.6188, -31.7871) (-24.6101, -31.7744) (-24.6015, -31.7617) (-24.593, -31.749) (-24.5845, -31.7363) (-24.5761, -31.7235) (-24.5678, -31.7108) (-24.5595, -31.698) (-24.5513, -31.6852) (-24.5432, -31.6724) (-24.5352, -31.6596) (-24.5272, -31.6467) (-24.5193, -31.6339) (-24.5115, -31.621) (-24.5038, -31.6081) (-24.4961, -31.5952) (-24.4885, -31.5823) (-24.481, -31.5693) (-24.4736, -31.5563) (-24.4662, -31.5434) (-24.459, -31.5304) (-24.4518, -31.5174) (-24.4446, -31.5043) (-24.4376, -31.4913) (-24.4306, -31.4782) (-24.4238, -31.4652) (-24.417, -31.4521) (-24.4103, -31.439) (-24.4036, -31.4259) (-24.3971, -31.4127) (-24.3906, -31.3996) (-24.3843, -31.3864) (-24.378, -31.3733) (-24.3718, -31.3601) (-24.3657, -31.3469) (-24.3597, -31.3337) (-24.3537, -31.3204) (-24.3479, -31.3072) (-24.3422, -31.2939) (-24.3365, -31.2806) (-24.331, -31.2674) (-24.3256, -31.2541) (-24.3202, -31.2408) (-24.3149, -31.2274) (-24.3098, -31.2141) (-24.3047, -31.2007) (-24.2998, -31.1874) (-24.295, -31.174) (-24.2903, -31.1606) (-24.2857, -31.1472) (-24.2812, -31.1338) (-24.2769, -31.1204) (-24.2726, -31.1069) (-24.2684, -31.0935) (-24.2644, -31.08) (-24.2605, -31.0666) (-24.2568, -31.0531) (-24.2533, -31.0396) (-24.25, -31.026) (-24.2468, -31.0125) (-24.2437, -30.999) (-24.2407, -30.9854) (-24.2379, -30.9719) (-24.2351, -30.9583) (-24.2327, -30.9447) (-24.2306, -30.9311) (-24.2293, -30.9202) (-24.2286, -30.912) (-24.2283, -30.9065) (-24.2282, -30.9038) knots -1 -1 -1 -1 -1 -1 -0.98571429 -0.97142857 -0.95714286 -0.94285714 -0.92857143 -0.91428571 -0.9 -0.88571429 -0.87142857 -0.85714286 -0.84285714 -0.82857143 -0.81428571 -0.8 -0.78571429 -0.77142857 -0.75714286 -0.74285714 -0.72857143 -0.71428571 -0.7 -0.68571429 -0.67142857 -0.65714286 -0.64285714 -0.62857143 -0.61428571 -0.6 -0.58571429 -0.57142857 -0.55714286 -0.54285714 -0.52857143 -0.51428571 -0.5 -0.48571429 -0.47142857 -0.45714286 -0.44285714 -0.42857143 -0.41428571 -0.4 -0.38571429 -0.37142857 -0.35714286 -0.34285714 -0.32857143 -0.31428571 -0.3 -0.28571429 -0.27142857 -0.25714286 -0.24285714 -0.22857143 -0.21428571 -0.2 -0.18571429 -0.17142857 -0.15714286 -0.14285714 -0.12857143 -0.11428571 -0.1 -0.08571429 -0.07142857 -0.05714286 -0.04285714 -0.02857143 -0.01428571 0 0 0 0 0 0 construction
  line L87 (-24.2282, -30.9038) -> (-24.2251, -30.8354) construction
  arc A164 (-23.9749, -30.5966) -> (-24.2251, -30.8354) centre (-23.9754, -30.8466) ccw construction
  arc A165 (-23.9749, -30.5966) -> (-23.8597, -30.5957) centre (-23.9648, -24.7074) ccw construction
  arc A166 (-23.6057, -30.8304) -> (-23.8597, -30.5957) centre (-23.8552, -30.8456) ccw construction
  line L88 (-23.6057, -30.8304) -> (-23.6015, -30.8987) construction
  spline S82 degree 5 poles (-23.6015, -30.8987) (-23.6013, -30.9015) (-23.6009, -30.9069) (-23.6001, -30.9151) (-23.5987, -30.926) (-23.5964, -30.9396) (-23.5937, -30.9531) (-23.5907, -30.9666) (-23.5876, -30.9801) (-23.5844, -30.9936) (-23.5812, -31.0071) (-23.5778, -31.0206) (-23.5742, -31.0341) (-23.5705, -31.0475) (-23.5665, -31.061) (-23.5624, -31.0744) (-23.5582, -31.0878) (-23.5538, -31.1011) (-23.5493, -31.1145) (-23.5447, -31.1279) (-23.5401, -31.1412) (-23.5353, -31.1545) (-23.5303, -31.1678) (-23.5253, -31.1811) (-23.5202, -31.1944) (-23.5149, -31.2077) (-23.5095, -31.2209) (-23.5041, -31.2342) (-23.4985, -31.2474) (-23.4928, -31.2606) (-23.4871, -31.2738) (-23.4812, -31.287) (-23.4753, -31.3001) (-23.4692, -31.3133) (-23.4631, -31.3264) (-23.4569, -31.3395) (-23.4506, -31.3526) (-23.4441, -31.3657) (-23.4377, -31.3788) (-23.4311, -31.3919) (-23.4244, -31.4049) (-23.4177, -31.4179) (-23.4108, -31.4309) (-23.4039, -31.4439) (-23.3969, -31.4569) (-23.3898, -31.4699) (-23.3826, -31.4828) (-23.3754, -31.4957) (-23.3681, -31.5086) (-23.3607, -31.5215) (-23.3532, -31.5344) (-23.3456, -31.5473) (-23.338, -31.5601) (-23.3303, -31.5729) (-23.3225, -31.5857) (-23.3146, -31.5985) (-23.3066, -31.6113) (-23.2986, -31.624) (-23.2905, -31.6368) (-23.2824, -31.6495) (-23.2741, -31.6622) (-23.2658, -31.6749) (-23.2574, -31.6875) (-23.249, -31.7002) (-23.2404, -31.7128) (-23.2318, -31.7254) (-23.2232, -31.738) (-23.2144, -31.7505) (-23.2056, -31.7631) (-23.1967, -31.7756) (-23.1878, -31.7881) (-23.1805, -31.7981) (-23.1751, -31.8056) (-23.1715, -31.8106) (-23.1696, -31.813) knots 0 0 0 0 0 0 0.01428571 0.02857143 0.04285714 0.05714286 0.07142857 0.08571429 0.1 0.11428571 0.12857143 0.14285714 0.15714286 0.17142857 0.18571429 0.2 0.21428571 0.22857143 0.24285714 0.25714286 0.27142857 0.28571429 0.3 0.31428571 0.32857143 0.34285714 0.35714286 0.37142857 0.38571429 0.4 0.41428571 0.42857143 0.44285714 0.45714286 0.47142857 0.48571429 0.5 0.51428571 0.52857143 0.54285714 0.55714286 0.57142857 0.58571429 0.6 0.61428571 0.62857143 0.64285714 0.65714286 0.67142857 0.68571429 0.7 0.71428571 0.72857143 0.74285714 0.75714286 0.77142857 0.78571429 0.8 0.81428571 0.82857143 0.84285714 0.85714286 0.87142857 0.88571429 0.9 0.91428571 0.92857143 0.94285714 0.95714286 0.97142857 0.98571429 1 1 1 1 1 1 construction
  arc A167 (-23.1696, -31.813) -> (-22.7799, -31.7585) centre (-23.9648, -24.7074) ccw construction
  spline S83 degree 5 poles (-22.7799, -31.7585) (-22.7788, -31.7556) (-22.7767, -31.7499) (-22.7735, -31.7412) (-22.7693, -31.7296) (-22.7641, -31.7151) (-22.759, -31.7006) (-22.754, -31.6861) (-22.749, -31.6717) (-22.7442, -31.6572) (-22.7393, -31.6427) (-22.7346, -31.6282) (-22.7299, -31.6137) (-22.7253, -31.5993) (-22.7208, -31.5848) (-22.7164, -31.5703) (-22.712, -31.5559) (-22.7077, -31.5414) (-22.7035, -31.5269) (-22.6994, -31.5125) (-22.6953, -31.498) (-22.6913, -31.4836) (-22.6874, -31.4691) (-22.6836, -31.4547) (-22.6799, -31.4402) (-22.6762, -31.4258) (-22.6726, -31.4114) (-22.6691, -31.3969) (-22.6657, -31.3825) (-22.6623, -31.3681) (-22.6591, -31.3537) (-22.6559, -31.3393) (-22.6528, -31.3249) (-22.6498, -31.3105) (-22.6469, -31.2962) (-22.6441, -31.2818) (-22.6413, -31.2674) (-22.6387, -31.2531) (-22.6361, -31.2387) (-22.6336, -31.2244) (-22.6312, -31.2101) (-22.6289, -31.1958) (-22.6267, -31.1815) (-22.6246, -31.1672) (-22.6226, -31.1529) (-22.6207, -31.1386) (-22.6189, -31.1244) (-22.6171, -31.1101) (-22.6155, -31.0959) (-22.614, -31.0817) (-22.6126, -31.0675) (-22.6113, -31.0533) (-22.6101, -31.0391) (-22.609, -31.025) (-22.608, -31.0108) (-22.6072, -30.9967) (-22.6064, -30.9826) (-22.6058, -30.9685) (-22.6052, -30.9545) (-22.6048, -30.9404) (-22.6046, -30.9264) (-22.6045, -30.9124) (-22.6046, -30.8985) (-22.6049, -30.8845) (-22.6053, -30.8706) (-22.6058, -30.8568) (-22.6065, -30.8429) (-22.6072, -30.8291) (-22.6081, -30.8153) (-22.6092, -30.8015) (-22.6107, -30.7879) (-22.6123, -30.777) (-22.6138, -30.7689) (-22.6149, -30.7635) (-22.6155, -30.7608) knots -1 -1 -1 -1 -1 -1 -0.98571429 -0.97142857 -0.95714286 -0.94285714 -0.92857143 -0.91428571 -0.9 -0.88571429 -0.87142857 -0.85714286 -0.84285714 -0.82857143 -0.81428571 -0.8 -0.78571429 -0.77142857 -0.75714286 -0.74285714 -0.72857143 -0.71428571 -0.7 -0.68571429 -0.67142857 -0.65714286 -0.64285714 -0.62857143 -0.61428571 -0.6 -0.58571429 -0.57142857 -0.55714286 -0.54285714 -0.52857143 -0.51428571 -0.5 -0.48571429 -0.47142857 -0.45714286 -0.44285714 -0.42857143 -0.41428571 -0.4 -0.38571429 -0.37142857 -0.35714286 -0.34285714 -0.32857143 -0.31428571 -0.3 -0.28571429 -0.27142857 -0.25714286 -0.24285714 -0.22857143 -0.21428571 -0.2 -0.18571429 -0.17142857 -0.15714286 -0.14285714 -0.12857143 -0.11428571 -0.1 -0.08571429 -0.07142857 -0.05714286 -0.04285714 -0.02857143 -0.01428571 0 0 0 0 0 0 construction
  line L89 (-22.6155, -30.7608) -> (-22.6302, -30.6939) construction
  arc A168 (-22.4503, -30.3985) -> (-22.6302, -30.6939) centre (-22.3861, -30.6401) ccw construction
  arc A169 (-22.4503, -30.3985) -> (-22.3393, -30.3678) centre (-23.9648, -24.7074) ccw construction
  arc A170 (-22.0332, -30.5288) -> (-22.3393, -30.3678) centre (-22.2703, -30.6081) ccw construction
  line L90 (-22.0332, -30.5288) -> (-22.0114, -30.5937) construction
  spline S84 degree 5 poles (-22.0114, -30.5937) (-22.0106, -30.5963) (-22.0088, -30.6015) (-22.0059, -30.6092) (-22.0017, -30.6194) (-21.9959, -30.6319) (-21.9898, -30.6443) (-21.9834, -30.6565) (-21.977, -30.6688) (-21.9704, -30.681) (-21.9637, -30.6932) (-21.957, -30.7053) (-21.95, -30.7174) (-21.943, -30.7294) (-21.9357, -30.7414) (-21.9283, -30.7533) (-21.9207, -30.7651) (-21.913, -30.7769) (-21.9052, -30.7887) (-21.8973, -30.8004) (-21.8893, -30.8121) (-21.8812, -30.8237) (-21.8731, -30.8353) (-21.8648, -30.8468) (-21.8563, -30.8583) (-21.8478, -30.8698) (-21.8392, -30.8812) (-21.8305, -30.8925) (-21.8217, -30.9039) (-21.8128, -30.9152) (-21.8038, -30.9264) (-21.7948, -30.9376) (-21.7856, -30.9488) (-21.7764, -30.96) (-21.7671, -30.971) (-21.7577, -30.9821) (-21.7482, -30.9931) (-21.7386, -31.0041) (-21.7289, -31.0151) (-21.7192, -31.026) (-21.7094, -31.0368) (-21.6995, -31.0477) (-21.6895, -31.0585) (-21.6795, -31.0692) (-21.6693, -31.0799) (-21.6591, -31.0906) (-21.6489, -31.1013) (-21.6385, -31.1119) (-21.6281, -31.1224) (-21.6176, -31.133) (-21.6071, -31.1435) (-21.5964, -31.1539) (-21.5857, -31.1644) (-21.5749, -31.1748) (-21.5641, -31.1851) (-21.5532, -31.1954) (-21.5422, -31.2057) (-21.5312, -31.2159) (-21.5201, -31.2261) (-21.5089, -31.2363) (-21.4976, -31.2464) (-21.4863, -31.2565) (-21.4749, -31.2666) (-21.4635, -31.2766) (-21.452, -31.2866) (-21.4404, -31.2965) (-21.4288, -31.3065) (-21.4171, -31.3163) (-21.4053, -31.3262) (-21.3935, -31.336) (-21.3816, -31.3457) (-21.3721, -31.3535) (-21.3649, -31.3593) (-21.3601, -31.3632) (-21.3576, -31.3651) knots 0 0 0 0 0 0 0.01428571 0.02857143 0.04285714 0.05714286 0.07142857 0.08571429 0.1 0.11428571 0.12857143 0.14285714 0.15714286 0.17142857 0.18571429 0.2 0.21428571 0.22857143 0.24285714 0.25714286 0.27142857 0.28571429 0.3 0.31428571 0.32857143 0.34285714 0.35714286 0.37142857 0.38571429 0.4 0.41428571 0.42857143 0.44285714 0.45714286 0.47142857 0.48571429 0.5 0.51428571 0.52857143 0.54285714 0.55714286 0.57142857 0.58571429 0.6 0.61428571 0.62857143 0.64285714 0.65714286 0.67142857 0.68571429 0.7 0.71428571 0.72857143 0.74285714 0.75714286 0.77142857 0.78571429 0.8 0.81428571 0.82857143 0.84285714 0.85714286 0.87142857 0.88571429 0.9 0.91428571 0.92857143 0.94285714 0.95714286 0.97142857 0.98571429 1 1 1 1 1 1 construction
  arc A171 (-21.3576, -31.3651) -> (-20.9953, -31.2116) centre (-23.9648, -24.7074) ccw construction
  spline S85 degree 5 poles (-20.9953, -31.2116) (-20.995, -31.2085) (-20.9945, -31.2024) (-20.9936, -31.1932) (-20.9926, -31.1809) (-20.9913, -31.1656) (-20.9901, -31.1503) (-20.989, -31.135) (-20.988, -31.1197) (-20.987, -31.1044) (-20.9861, -31.0892) (-20.9853, -31.074) (-20.9845, -31.0588) (-20.9838, -31.0436) (-20.9832, -31.0285) (-20.9827, -31.0134) (-20.9822, -30.9983) (-20.9818, -30.9832) (-20.9815, -30.9681) (-20.9812, -30.9531) (-20.981, -30.9381) (-20.9809, -30.9231) (-20.9809, -30.9081) (-20.9809, -30.8932) (-20.9811, -30.8783) (-20.9813, -30.8634) (-20.9815, -30.8485) (-20.9819, -30.8337) (-20.9823, -30.8188) (-20.9828, -30.8041) (-20.9834, -30.7893) (-20.984, -30.7746) (-20.9848, -30.7599) (-20.9856, -30.7452) (-20.9865, -30.7306) (-20.9875, -30.7159) (-20.9886, -30.7014) (-20.9897, -30.6868) (-20.9909, -30.6723) (-20.9922, -30.6578) (-20.9936, -30.6434) (-20.9951, -30.6289) (-20.9967, -30.6146) (-20.9984, -30.6002) (-21.0001, -30.5859) (-21.002, -30.5716) (-21.0039, -30.5574) (-21.0059, -30.5432) (-21.008, -30.529) (-21.0102, -30.5149) (-21.0125, -30.5008) (-21.0149, -30.4868) (-21.0175, -30.4728) (-21.0201, -30.4588) (-21.0228, -30.4449) (-21.0256, -30.4311) (-21.0286, -30.4172) (-21.0316, -30.4035) (-21.0347, -30.3897) (-21.0379, -30.3761) (-21.0413, -30.3625) (-21.0449, -30.3489) (-21.0486, -30.3355) (-21.0524, -30.3221) (-21.0564, -30.3088) (-21.0606, -30.2955) (-21.0648, -30.2823) (-21.0691, -30.2691) (-21.0735, -30.256) (-21.0781, -30.243) (-21.0831, -30.2302) (-21.0874, -30.2201) (-21.091, -30.2127) (-21.0934, -30.2078) (-21.0947, -30.2053) knots -1 -1 -1 -1 -1 -1 -0.98571429 -0.97142857 -0.95714286 -0.94285714 -0.92857143 -0.91428571 -0.9 -0.88571429 -0.87142857 -0.85714286 -0.84285714 -0.82857143 -0.81428571 -0.8 -0.78571429 -0.77142857 -0.75714286 -0.74285714 -0.72857143 -0.71428571 -0.7 -0.68571429 -0.67142857 -0.65714286 -0.64285714 -0.62857143 -0.61428571 -0.6 -0.58571429 -0.57142857 -0.55714286 -0.54285714 -0.52857143 -0.51428571 -0.5 -0.48571429 -0.47142857 -0.45714286 -0.44285714 -0.42857143 -0.41428571 -0.4 -0.38571429 -0.37142857 -0.35714286 -0.34285714 -0.32857143 -0.31428571 -0.3 -0.28571429 -0.27142857 -0.25714286 -0.24285714 -0.22857143 -0.21428571 -0.2 -0.18571429 -0.17142857 -0.15714286 -0.14285714 -0.12857143 -0.11428571 -0.1 -0.08571429 -0.07142857 -0.05714286 -0.04285714 -0.02857143 -0.01428571 0 0 0 0 0 0 construction
  line L91 (-21.0947, -30.2053) -> (-21.1262, -30.1445) construction
  arc A172 (-21.029, -29.8127) -> (-21.1262, -30.1445) centre (-20.9043, -30.0294) ccw construction
  arc A173 (-21.029, -29.8127) -> (-20.9296, -29.7542) centre (-23.9648, -24.7074) ccw construction
  arc A174 (-20.5923, -29.8305) -> (-20.9296, -29.7542) centre (-20.8008, -29.9685) ccw construction
  line L92 (-20.5923, -29.8305) -> (-20.5545, -29.8876) construction
  spline S86 degree 5 poles (-20.5545, -29.8876) (-20.553, -29.8899) (-20.5499, -29.8944) (-20.5451, -29.9011) (-20.5384, -29.9099) (-20.5296, -29.9204) (-20.5205, -29.9308) (-20.5112, -29.941) (-20.5018, -29.9512) (-20.4923, -29.9613) (-20.4827, -29.9713) (-20.473, -29.9813) (-20.4632, -29.9912) (-20.4532, -30.001) (-20.4431, -30.0106) (-20.4329, -30.0202) (-20.4225, -30.0297) (-20.412, -30.0391) (-20.4014, -30.0484) (-20.3908, -30.0577) (-20.3801, -30.0669) (-20.3692, -30.076) (-20.3583, -30.0851) (-20.3473, -30.0941) (-20.3362, -30.103) (-20.325, -30.1119) (-20.3138, -30.1207) (-20.3024, -30.1294) (-20.291, -30.1381) (-20.2795, -30.1467) (-20.2679, -30.1552) (-20.2562, -30.1637) (-20.2445, -30.1721) (-20.2327, -30.1805) (-20.2208, -30.1888) (-20.2088, -30.1971) (-20.1968, -30.2052) (-20.1847, -30.2134) (-20.1726, -30.2214) (-20.1603, -30.2295) (-20.148, -30.2374) (-20.1357, -30.2453) (-20.1233, -30.2532) (-20.1108, -30.261) (-20.0982, -30.2687) (-20.0856, -30.2764) (-20.0729, -30.284) (-20.0602, -30.2916) (-20.0474, -30.2991) (-20.0345, -30.3066) (-20.0216, -30.314) (-20.0086, -30.3213) (-19.9956, -30.3286) (-19.9825, -30.3359) (-19.9694, -30.343) (-19.9561, -30.3502) (-19.9429, -30.3573) (-19.9296, -30.3643) (-19.9162, -30.3713) (-19.9027, -30.3782) (-19.8893, -30.3851) (-19.8757, -30.3919) (-19.8621, -30.3987) (-19.8485, -30.4054) (-19.8348, -30.4121) (-19.821, -30.4187) (-19.8072, -30.4252) (-19.7934, -30.4317) (-19.7795, -30.4382) (-19.7655, -30.4446) (-19.7515, -30.451) (-19.7403, -30.456) (-19.7318, -30.4598) (-19.7262, -30.4623) (-19.7233, -30.4635) knots 0 0 0 0 0 0 0.01428571 0.02857143 0.04285714 0.05714286 0.07142857 0.08571429 0.1 0.11428571 0.12857143 0.14285714 0.15714286 0.17142857 0.18571429 0.2 0.21428571 0.22857143 0.24285714 0.25714286 0.27142857 0.28571429 0.3 0.31428571 0.32857143 0.34285714 0.35714286 0.37142857 0.38571429 0.4 0.41428571 0.42857143 0.44285714 0.45714286 0.47142857 0.48571429 0.5 0.51428571 0.52857143 0.54285714 0.55714286 0.57142857 0.58571429 0.6 0.61428571 0.62857143 0.64285714 0.65714286 0.67142857 0.68571429 0.7 0.71428571 0.72857143 0.74285714 0.75714286 0.77142857 0.78571429 0.8 0.81428571 0.82857143 0.84285714 0.85714286 0.87142857 0.88571429 0.9 0.91428571 0.92857143 0.94285714 0.95714286 0.97142857 0.98571429 1 1 1 1 1 1 construction
  arc A175 (-19.7233, -30.4635) -> (-19.4131, -30.2214) centre (-23.9648, -24.7074) ccw construction
  spline S87 degree 5 poles (-19.4131, -30.2214) (-19.4136, -30.2184) (-19.4147, -30.2123) (-19.4162, -30.2032) (-19.4184, -30.1911) (-19.4212, -30.1759) (-19.424, -30.1608) (-19.4269, -30.1458) (-19.4298, -30.1308) (-19.4328, -30.1158) (-19.4359, -30.1008) (-19.439, -30.0859) (-19.4422, -30.071) (-19.4455, -30.0562) (-19.4488, -30.0414) (-19.4522, -30.0267) (-19.4556, -30.012) (-19.4591, -29.9973) (-19.4627, -29.9827) (-19.4664, -29.9681) (-19.4701, -29.9535) (-19.4739, -29.939) (-19.4777, -29.9245) (-19.4816, -29.9101) (-19.4856, -29.8957) (-19.4896, -29.8814) (-19.4937, -29.8671) (-19.4979, -29.8529) (-19.5022, -29.8387) (-19.5065, -29.8245) (-19.5109, -29.8104) (-19.5153, -29.7964) (-19.5198, -29.7824) (-19.5244, -29.7684) (-19.5291, -29.7545) (-19.5338, -29.7406) (-19.5386, -29.7268) (-19.5435, -29.7131) (-19.5484, -29.6994) (-19.5534, -29.6857) (-19.5585, -29.6721) (-19.5637, -29.6586) (-19.5689, -29.6451) (-19.5743, -29.6316) (-19.5797, -29.6183) (-19.5851, -29.605) (-19.5907, -29.5917) (-19.5963, -29.5785) (-19.602, -29.5654) (-19.6078, -29.5523) (-19.6137, -29.5393) (-19.6196, -29.5264) (-19.6257, -29.5135) (-19.6318, -29.5007) (-19.6381, -29.488) (-19.6444, -29.4753) (-19.6508, -29.4627) (-19.6573, -29.4502) (-19.6638, -29.4378) (-19.6705, -29.4254) (-19.6773, -29.4131) (-19.6842, -29.401) (-19.6913, -29.3889) (-19.6985, -29.377) (-19.7058, -29.3652) (-19.7132, -29.3534) (-19.7207, -29.3418) (-19.7282, -29.3302) (-19.7359, -29.3186) (-19.7437, -29.3073) (-19.7519, -29.2962) (-19.7587, -29.2876) (-19.764, -29.2813) (-19.7677, -29.2772) (-19.7695, -29.2752) knots -1 -1 -1 -1 -1 -1 -0.98571429 -0.97142857 -0.95714286 -0.94285714 -0.92857143 -0.91428571 -0.9 -0.88571429 -0.87142857 -0.85714286 -0.84285714 -0.82857143 -0.81428571 -0.8 -0.78571429 -0.77142857 -0.75714286 -0.74285714 -0.72857143 -0.71428571 -0.7 -0.68571429 -0.67142857 -0.65714286 -0.64285714 -0.62857143 -0.61428571 -0.6 -0.58571429 -0.57142857 -0.55714286 -0.54285714 -0.52857143 -0.51428571 -0.5 -0.48571429 -0.47142857 -0.45714286 -0.44285714 -0.42857143 -0.41428571 -0.4 -0.38571429 -0.37142857 -0.35714286 -0.34285714 -0.32857143 -0.31428571 -0.3 -0.28571429 -0.27142857 -0.25714286 -0.24285714 -0.22857143 -0.21428571 -0.2 -0.18571429 -0.17142857 -0.15714286 -0.14285714 -0.12857143 -0.11428571 -0.1 -0.08571429 -0.07142857 -0.05714286 -0.04285714 -0.02857143 -0.01428571 0 0 0 0 0 0 construction
  line L93 (-19.7695, -29.2752) -> (-19.8157, -29.2246) construction
  arc A176 (-19.8077, -28.8789) -> (-19.8157, -29.2246) centre (-19.6312, -29.0559) ccw construction
  arc A177 (-19.8077, -28.8789) -> (-19.7268, -28.7967) centre (-23.9648, -24.7074) ccw construction
  arc A178 (-19.3813, -28.7831) -> (-19.7268, -28.7967) centre (-19.5469, -28.9703) ccw construction
  line L94 (-19.3813, -28.7831) -> (-19.33, -28.8285) construction